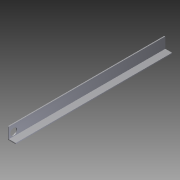
# Autodesk Inventor part: manipulator L frame left
Saved by Autodesk Inventor 2012 (Build 160160000, 160)
## iProperties
Created: 2013-09-01
Part Number: manipulator L frame left
Material: Default
Document SubType Name: Modeling
Designer: Bryce
Density: 1 g/cm^3
Author: Bryce
Autodesk Inventor part; units mm, degrees
ref_plane "YZ Plane" through (0, 0, 0) normal (1, 0, 0) x (0, 1, 0)
ref_plane "XZ Plane" through (0, 0, 0) normal (0, 1, 0) x (-1, 0, 0)
ref_plane "XY Plane" through (0, 0, 0) normal (0, 0, 1) x (1, 0, 0)
sketch "Sketch1" plane through (0, 0, 0) normal (0, 0, 1) x (1, 0, 0)
  line L0 (0, 0) -> (25.4, 0)
  line L1 (25.4, 0) -> (25.4, 3.175)
  line L2 (3.175, 38.1) -> (0, 38.1)
  line L3 (0, 38.1) -> (0, 0)
  line L4 (3.175, 38.1) -> (3.175, 3.175)
  line L5 (3.175, 3.175) -> (25.4, 3.175)
  dimension "d0" = 38.1
  dimension "d1" = 25.4
  dimension "d2" = 3.175
  dimension "d3" = 3.175
  constraints: 12 end point, 2 parallel, 1 horizontal, 1 perpendicular
  measures "d0" distance of L2.end L0.start
  measures "d1" distance of L0.start L0.end
  measures "d2" distance between parallel lines of L4 L3
  measures "d3" distance between parallel lines of L5 L0
extrude "Extrusion1" add sketch "Sketch1" along normal blind 508
sketch "Sketch2" plane through (0, 0, 0) normal (-1, 0, 0) x (0, 0, 1)
  line L0 (508, 0) -> (508, 38.1) projected
  line L1 (0, 0) -> (508, 0) projected
  circle A0 centre (492.125, 15.875) radius 11.1125
  arc A1 (492.125, 0) -> (508, 15.875) centre (492.125, 15.875) ccw
  dimension "d6" = 22.225
  dimension "d7" = 15.875
  dimension "d8" = 15.875
  constraints: 2 centre point, 2 point on circle, 2 point on line, 1 coincident, 1 tangent
  measures "d6" diameter of A0
  measures "d7" distance from line of L1 A0.centre
  measures "d8" distance from line of L0 A0.centre
extrude "Extrusion2" cut sketch "Sketch2" against normal blind 508 contours A0
equation "\"d3\" = d2"
equation "\"d8\" = d7"
body "Solid1"
